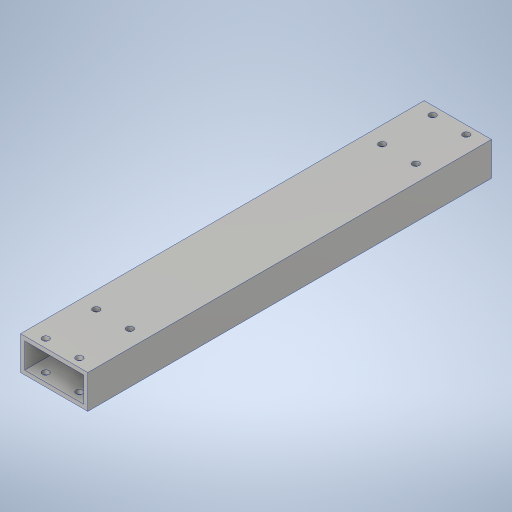
# Autodesk Inventor part: GP1-003
Saved by Autodesk Inventor 2023.4 (Build 274418000, 418)
## iProperties
Created: 2025-01-07
Part Number: GP1-003
Material: Aluminum 6061
Document SubType Name: Modeling
Designer: mavericks
Density: 2.7 g/cm^3
Appearance: Aluminum - Flat
Author: mavericks
Autodesk Inventor part; units mm, degrees
ref_plane "YZ Plane" through (0, 0, 0) normal (1, 0, 0) x (0, 1, 0)
ref_plane "XZ Plane" through (0, 0, 0) normal (0, 1, 0) x (-1, 0, 0)
ref_plane "XY Plane" through (0, 0, 0) normal (0, 0, 1) x (1, 0, 0)
sketch "Sketch1" plane through (0, 0, 0) normal (0, 0, 1) x (1, 0, 0)
  line L0 (-25.4, 12.7) -> (25.4, 12.7)
  line L1 (25.4, 12.7) -> (25.4, -12.7)
  line L2 (25.4, -12.7) -> (-25.4, -12.7)
  line L3 (-25.4, -12.7) -> (-25.4, 12.7)
  line L4 (-25.4, 12.7) -> (25.4, -12.7) construction
  line L5 (25.4, 12.7) -> (-25.4, -12.7) construction
  line L6 (22.225, 9.525) -> (-22.225, 9.525)
  line L7 (-22.225, 9.525) -> (-22.225, -9.525)
  line L8 (-22.225, -9.525) -> (22.225, -9.525)
  line L9 (22.225, -9.525) -> (22.225, 9.525)
  line L10 (22.225, 9.525) -> (-22.225, -9.525) construction
  line L11 (-22.225, 9.525) -> (22.225, -9.525) construction
  point P0 (0, 0)
  dimension "d0" = 50.8
  dimension "d1" = 25.4
  dimension "d2" = 3.175
  dimension "d3" = 3.175
  constraints: 24 end point, 4 midpoint, 4 parallel, 2 horizontal, 2 perpendicular
  measures "d0" distance of L1.end L2.end
  measures "d1" distance of L2.end L0.start
  measures "d2" distance between parallel lines of L7 L3
  measures "d3" distance between parallel lines of L2 L8
extrude "Extrusion1" add sketch "Sketch1" along normal mid plane 304.8
sketch "Sketch2" plane through (-25.4, 12.7, 152.4) normal (0, 1, 0) x (1, 0, 0)
  line L0 (50.8, 0) -> (0, 0) projected
  line L1 (0, 304.8) -> (50.8, 304.8) projected
  line L2 (0, 304.8) -> (0, 0) projected
  line L3 (50.8, 304.8) -> (50.8, 0) projected
  point P0 (25.4, 152.4)
  point P1 (12.7, 6.35)
  point P2 (38.1, 6.35)
  point P3 (38.1, 44.45)
  point P4 (12.7, 44.45)
  point P5 (12.7, 298.45)
  point P6 (38.1, 298.45)
  point P7 (38.1, 260.35)
  point P8 (12.7, 260.35)
  dimension "d6" = 6.35
  dimension "d7" = 25.4
  dimension "d8" = 38.1
  dimension "d9" = 6.35
  dimension "d10" = 12.7
  dimension "d11" = 12.7
  dimension "d12" = 12.7
  dimension "d13" = 38.1
  constraints: 6 vertical alignment, 4 horizontal alignment
  measures "d6" distance from line of L0 point (12.7, 6.35)
  measures "d7" distance of point (12.7, 6.35) point (38.1, 6.35)
  measures "d8" distance of point (12.7, 44.45) point (12.7, 6.35)
  measures "d9" distance from line of L1 point (38.1, 298.45)
  measures "d10" distance from line of L2 point (12.7, 44.45)
  measures "d11" distance from line of point (38.1, 44.45) L3
  measures "d12" distance from line of L3 point (38.1, 260.35)
  measures "d13" distance of point (12.7, 298.45) point (12.7, 260.35)
hole "Hole1" at (-12.7, 12.7, 146.05) at (12.7, 12.7, 146.05) at (12.7, 12.7, 107.95) at (-12.7, 12.7, 107.95) at (-12.7, 12.7, -146.05) at (12.7, 12.7, -146.05) at (12.7, 12.7, -107.95) at (-12.7, 12.7, -107.95) direction (0, -1, 0) diameter 5.1054 end through all clearance for "Flat Head Machine Screw (82)" size "#10" standard "Ansi Unified Screw Threads"
body "Solid1"
